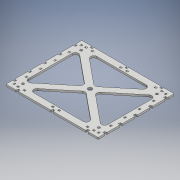
# Autodesk Inventor part: turtlebot_installation_top
Saved by Autodesk Inventor 2018 (Build 220112000, 112)
## iProperties
Created: 2018-07-16
Part Number: turtlebot_installation_top
Material: Generic
Document SubType Name: Modeling
Designer: Tsche
Density: 1 g/cm^3
Appearance: Default
Author: Tsche
Autodesk Inventor part; units mm, degrees
ref_plane "YZ Plane" through (0, 0, 0) normal (1, 0, 0) x (0, 1, 0)
ref_plane "XZ Plane" through (0, 0, 0) normal (0, 1, 0) x (-1, 0, 0)
ref_plane "XY Plane" through (0, 0, 0) normal (0, 0, 1) x (1, 0, 0)
sketch "Sketch1" plane through (0, 0, 0) normal (0, 0, 1) x (1, 0, 0)
  line L0 (-73, 60) -> (-73, 49.6)
  line L1 (-73, -60) -> (0, 0) construction
  line L2 (-73, -1.6) -> (-69.9, -1.6)
  line L3 (-69.9, -1.6) -> (-69.9, 1.6)
  line L4 (-69.9, 1.6) -> (-73, 1.6)
  line L5 (-73, 1.6) -> (-73, -1.6) construction
  line L6 (-73, -1.6) -> (-73, -22.4)
  line L7 (-73, 0) -> (-69.9, 0) construction
  line L8 (-102.2, 0) -> (102.2, 0) construction
  line L9 (0, 84) -> (0, -84) construction
  line L10 (-73, -25.6) -> (-69.9, -25.6)
  line L11 (-69.9, -25.6) -> (-69.9, -22.4)
  line L12 (-69.9, -22.4) -> (-73, -22.4)
  line L13 (-73, 49.6) -> (-69.9, 49.6)
  line L14 (-69.9, 49.6) -> (-69.9, 46.4)
  line L15 (-69.9, 46.4) -> (-73, 46.4)
  line L16 (-73, 49.6) -> (-73, 46.4) construction
  line L17 (-73, 46.4) -> (-73, 25.6)
  line L18 (-73, -22.4) -> (-73, -25.6) construction
  line L19 (-73, -25.6) -> (-73, -46.4)
  line L20 (-73, -24) -> (-69.9, -24) construction
  line L21 (-73, 48) -> (-69.9, 48) construction
  line L22 (-73, -49.6) -> (-69.9, -49.6)
  line L23 (-69.9, -49.6) -> (-69.9, -46.4)
  line L24 (-69.9, -46.4) -> (-73, -46.4)
  line L25 (-73, -46.4) -> (-73, -49.6) construction
  line L26 (-73, -49.6) -> (-73, -60)
  line L27 (-73, -48) -> (-69.9, -48) construction
  line L28 (-73, 22.4) -> (-69.9, 22.4)
  line L29 (-69.9, 22.4) -> (-69.9, 25.6)
  line L30 (-69.9, 25.6) -> (-73, 25.6)
  line L31 (-73, 25.6) -> (-73, 22.4) construction
  line L32 (-73, 22.4) -> (-73, 1.6)
  line L33 (-73, 24) -> (-69.9, 24) construction
  line L34 (0, 60) -> (-1.5, 60) construction
  line L35 (0, 0) -> (-73, 60) construction
  line L36 (-67, -10) -> (-65.7, -10)
  line L37 (-65.7, -10) -> (-65.7, -13)
  line L38 (-65.7, -13) -> (-67, -13)
  line L39 (-67, -13) -> (-67, -10)
  line L40 (-67, -11.5) -> (-65.7, -11.5) construction
  line L41 (-65.7, -35.5) -> (-67, -35.5)
  line L42 (-67, -34) -> (-65.7, -34) construction
  line L43 (-67, -35.5) -> (-67, -32.5)
  line L44 (-67, -32.5) -> (-65.7, -32.5)
  line L45 (-65.7, -32.5) -> (-65.7, -35.5)
  line L46 (-67, -51.5) -> (-65.7, -51.5)
  line L47 (-67, -53) -> (-65.7, -53) construction
  line L48 (-65.7, -51.5) -> (-65.7, -54.5)
  line L49 (-67, -54.5) -> (-67, -51.5)
  line L50 (-65.7, -54.5) -> (-67, -54.5)
  line L51 (-67, 10) -> (-65.7, 10)
  line L52 (-65.7, 10) -> (-65.7, 13)
  line L53 (-65.7, 13) -> (-67, 13)
  line L54 (-67, 13) -> (-67, 10)
  line L55 (-67, 11.5) -> (-65.7, 11.5) construction
  line L56 (-65.7, 35.5) -> (-67, 35.5)
  line L57 (-67, 34) -> (-65.7, 34) construction
  line L58 (-67, 35.5) -> (-67, 32.5)
  line L59 (-67, 32.5) -> (-65.7, 32.5)
  line L60 (-65.7, 32.5) -> (-65.7, 35.5)
  line L61 (-67, 51.5) -> (-65.7, 51.5)
  line L62 (-67, 53) -> (-65.7, 53) construction
  line L63 (-65.7, 51.5) -> (-65.7, 54.5)
  line L64 (-67, 54.5) -> (-67, 51.5)
  line L65 (-65.7, 54.5) -> (-67, 54.5)
  line L66 (73, 60) -> (73, 49.6)
  line L67 (73, -60) -> (0, 0) construction
  line L68 (73, -1.6) -> (69.9, -1.6)
  line L69 (69.9, -1.6) -> (69.9, 1.6)
  line L70 (69.9, 1.6) -> (73, 1.6)
  line L71 (73, 1.6) -> (73, -1.6) construction
  line L72 (73, -1.6) -> (73, -22.4)
  line L73 (73, 0) -> (69.9, 0) construction
  line L74 (73, -25.6) -> (69.9, -25.6)
  line L75 (69.9, -25.6) -> (69.9, -22.4)
  line L76 (69.9, -22.4) -> (73, -22.4)
  line L77 (73, 49.6) -> (69.9, 49.6)
  line L78 (69.9, 49.6) -> (69.9, 46.4)
  line L79 (69.9, 46.4) -> (73, 46.4)
  line L80 (73, 49.6) -> (73, 46.4) construction
  line L81 (73, 46.4) -> (73, 25.6)
  line L82 (73, -22.4) -> (73, -25.6) construction
  line L83 (73, -25.6) -> (73, -46.4)
  line L84 (73, -24) -> (69.9, -24) construction
  line L85 (73, 48) -> (69.9, 48) construction
  line L86 (73, -49.6) -> (69.9, -49.6)
  line L87 (69.9, -49.6) -> (69.9, -46.4)
  line L88 (69.9, -46.4) -> (73, -46.4)
  line L89 (73, -46.4) -> (73, -49.6) construction
  line L90 (73, -49.6) -> (73, -60)
  line L91 (73, -48) -> (69.9, -48) construction
  line L92 (73, 22.4) -> (69.9, 22.4)
  line L93 (69.9, 22.4) -> (69.9, 25.6)
  line L94 (69.9, 25.6) -> (73, 25.6)
  line L95 (73, 25.6) -> (73, 22.4) construction
  line L96 (73, 22.4) -> (73, 1.6)
  line L97 (73, 24) -> (69.9, 24) construction
  line L98 (0, 0) -> (73, 60) construction
  line L99 (67, -10) -> (65.7, -10)
  line L100 (65.7, -10) -> (65.7, -13)
  line L101 (65.7, -13) -> (67, -13)
  line L102 (67, -13) -> (67, -10)
  line L103 (67, -11.5) -> (65.7, -11.5) construction
  line L104 (65.7, -35.5) -> (67, -35.5)
  line L105 (67, -34) -> (65.7, -34) construction
  line L106 (67, -35.5) -> (67, -32.5)
  line L107 (67, -32.5) -> (65.7, -32.5)
  line L108 (65.7, -32.5) -> (65.7, -35.5)
  line L109 (67, -51.5) -> (65.7, -51.5)
  line L110 (67, -53) -> (65.7, -53) construction
  line L111 (65.7, -51.5) -> (65.7, -54.5)
  line L112 (67, -54.5) -> (67, -51.5)
  line L113 (65.7, -54.5) -> (67, -54.5)
  line L114 (67, 10) -> (65.7, 10)
  line L115 (67, 11.5) -> (65.7, 11.5) construction
  line L116 (67, 13) -> (67, 10)
  line L117 (65.7, 10) -> (65.7, 13)
  line L118 (65.7, 13) -> (67, 13)
  line L119 (67, 51.5) -> (65.7, 51.5)
  line L120 (67, 53) -> (65.7, 53) construction
  line L121 (67, 54.5) -> (67, 51.5)
  line L122 (65.7, 51.5) -> (65.7, 54.5)
  line L123 (65.7, 54.5) -> (67, 54.5)
  line L124 (67, 32.5) -> (65.7, 32.5)
  line L125 (67, 34) -> (65.7, 34) construction
  line L126 (67, 35.5) -> (67, 32.5)
  line L127 (65.7, 32.5) -> (65.7, 35.5)
  line L128 (65.7, 35.5) -> (67, 35.5)
  line L129 (-63, 45.3087) -> (-63, -45.3087)
  line L130 (-63, -45.3087) -> (-7.8744, 0)
  line L131 (-63, 45.3087) -> (-7.8744, 0)
  line L132 (-52.9589, 50) -> (0, 6.4721)
  line L133 (52.9589, 50) -> (0, 6.4721)
  line L134 (-52.9589, 50) -> (52.9589, 50)
  line L135 (63, 45.3087) -> (63, -45.3087)
  line L136 (63, -45.3087) -> (7.8744, 0)
  line L137 (63, 45.3087) -> (7.8744, 0)
  line L138 (-52.9589, -50) -> (0, -6.4721)
  line L139 (52.9589, -50) -> (0, -6.4721)
  line L140 (-52.9589, -50) -> (52.9589, -50)
  line L141 (-1.5, 60) -> (-1.5, 56.9)
  line L142 (-1.5, 56.9) -> (0, 56.9)
  line L143 (-1.5, 60) -> (-53.4, 60)
  line L144 (-56.6, 60) -> (-56.6, 56.9)
  line L145 (-56.6, 56.9) -> (-53.4, 56.9)
  line L146 (-53.4, 56.9) -> (-53.4, 60)
  line L147 (-56.6, 60) -> (-73, 60)
  line L148 (-53.4, 60) -> (-56.6, 60) construction
  line L149 (-55, 56.9) -> (-55, 60) construction
  line L150 (-3.5, 54) -> (-6.5, 54)
  line L151 (-6.5, 54) -> (-6.5, 52.7)
  line L152 (-6.5, 52.7) -> (-3.5, 52.7)
  line L153 (-3.5, 52.7) -> (-3.5, 54)
  line L154 (-5, 54) -> (-5, 52.7) construction
  line L155 (-48.5, 52.7) -> (-48.5, 54)
  line L156 (-50, 54) -> (-50, 52.7) construction
  line L157 (-51.5, 54) -> (-51.5, 52.7)
  line L158 (-48.5, 54) -> (-51.5, 54)
  line L159 (-51.5, 52.7) -> (-48.5, 52.7)
  line L160 (-61.5, 52.7) -> (-61.5, 54)
  line L161 (-60, 54) -> (-60, 52.7) construction
  line L162 (-58.5, 54) -> (-58.5, 52.7)
  line L163 (-61.5, 54) -> (-58.5, 54)
  line L164 (-58.5, 52.7) -> (-61.5, 52.7)
  line L165 (0, -60) -> (-1.5, -60) construction
  line L166 (-1.5, -60) -> (-1.5, -56.9)
  line L167 (-1.5, -56.9) -> (0, -56.9)
  line L168 (-1.5, -60) -> (-53.4, -60)
  line L169 (-56.6, -60) -> (-56.6, -56.9)
  line L170 (-56.6, -56.9) -> (-53.4, -56.9)
  line L171 (-53.4, -56.9) -> (-53.4, -60)
  line L172 (-56.6, -60) -> (-73, -60)
  line L173 (-53.4, -60) -> (-56.6, -60) construction
  line L174 (-55, -56.9) -> (-55, -60) construction
  line L175 (-3.5, -54) -> (-6.5, -54)
  line L176 (-6.5, -54) -> (-6.5, -52.7)
  line L177 (-6.5, -52.7) -> (-3.5, -52.7)
  line L178 (-3.5, -52.7) -> (-3.5, -54)
  line L179 (-5, -54) -> (-5, -52.7) construction
  line L180 (-48.5, -52.7) -> (-48.5, -54)
  line L181 (-50, -54) -> (-50, -52.7) construction
  line L182 (-51.5, -54) -> (-51.5, -52.7)
  line L183 (-48.5, -54) -> (-51.5, -54)
  line L184 (-51.5, -52.7) -> (-48.5, -52.7)
  line L185 (-58.5, -54) -> (-58.5, -52.7)
  line L186 (-60, -54) -> (-60, -52.7) construction
  line L187 (-58.5, -52.7) -> (-61.5, -52.7)
  line L188 (-61.5, -52.7) -> (-61.5, -54)
  line L189 (-61.5, -54) -> (-58.5, -54)
  line L190 (0, -60) -> (1.5, -60) construction
  line L191 (61.5, -52.7) -> (61.5, -54)
  line L192 (58.5, -52.7) -> (61.5, -52.7)
  line L193 (60, -54) -> (60, -52.7) construction
  line L194 (58.5, -54) -> (58.5, -52.7)
  line L195 (56.6, -60) -> (73, -60)
  line L196 (61.5, -54) -> (58.5, -54)
  line L197 (6.5, -52.7) -> (3.5, -52.7)
  line L198 (3.5, -52.7) -> (3.5, -54)
  line L199 (5, -54) -> (5, -52.7) construction
  line L200 (6.5, -54) -> (6.5, -52.7)
  line L201 (3.5, -54) -> (6.5, -54)
  line L202 (1.5, -56.9) -> (0, -56.9)
  line L203 (1.5, -60) -> (1.5, -56.9)
  line L204 (1.5, -60) -> (53.4, -60)
  line L205 (56.6, -60) -> (56.6, -56.9)
  line L206 (55, -56.9) -> (55, -60) construction
  line L207 (56.6, -56.9) -> (53.4, -56.9)
  line L208 (53.4, -60) -> (56.6, -60) construction
  line L209 (51.5, -54) -> (51.5, -52.7)
  line L210 (50, -54) -> (50, -52.7) construction
  line L211 (48.5, -52.7) -> (48.5, -54)
  line L212 (51.5, -52.7) -> (48.5, -52.7)
  line L213 (48.5, -54) -> (51.5, -54)
  line L214 (53.4, -56.9) -> (53.4, -60)
  line L215 (0, 60) -> (1.5, 60) construction
  line L216 (1.5, 60) -> (1.5, 56.9)
  line L217 (1.5, 56.9) -> (0, 56.9)
  line L218 (1.5, 60) -> (53.4, 60)
  line L219 (56.6, 60) -> (56.6, 56.9)
  line L220 (56.6, 56.9) -> (53.4, 56.9)
  line L221 (53.4, 56.9) -> (53.4, 60)
  line L222 (56.6, 60) -> (73, 60)
  line L223 (53.4, 60) -> (56.6, 60) construction
  line L224 (55, 56.9) -> (55, 60) construction
  line L225 (3.5, 54) -> (6.5, 54)
  line L226 (6.5, 54) -> (6.5, 52.7)
  line L227 (6.5, 52.7) -> (3.5, 52.7)
  line L228 (3.5, 52.7) -> (3.5, 54)
  line L229 (5, 54) -> (5, 52.7) construction
  line L230 (48.5, 52.7) -> (48.5, 54)
  line L231 (50, 54) -> (50, 52.7) construction
  line L232 (51.5, 54) -> (51.5, 52.7)
  line L233 (48.5, 54) -> (51.5, 54)
  line L234 (51.5, 52.7) -> (48.5, 52.7)
  line L235 (58.5, 54) -> (58.5, 52.7)
  line L236 (60, 54) -> (60, 52.7) construction
  line L237 (58.5, 52.7) -> (61.5, 52.7)
  line L238 (61.5, 52.7) -> (61.5, 54)
  line L239 (61.5, 54) -> (58.5, 54)
  circle A0 centre (0, 0) radius 3.15
  circle A1 centre (-60, -46) radius 1.85
  circle A2 centre (60, -46) radius 1.85
  circle A3 centre (-60, 46) radius 1.85
  circle A4 centre (60, 46) radius 1.85
  dimension "d0" = 120
  dimension "d2" = 3.1
  dimension "d3" = 3.2
  dimension "d4" = 24
  dimension "d5" = 24
  dimension "d6" = 24
  dimension "d7" = 24
  dimension "d8" = 73
  dimension "d9" = 3
  dimension "d10" = 1.3
  dimension "d11" = 11.5
  dimension "d12" = 6
  dimension "d15" = 22.5
  dimension "d22" = 41.5
  dimension "d33" = 10
  dimension "d34" = 5
  dimension "d35" = 5
  dimension "d36" = 5
  dimension "d37" = 10
  dimension "d38" = 10
  dimension "d39" = 1.5
  dimension "d40" = 18
  dimension "d41" = 6
  dimension "d42" = 5
  dimension "d45" = 45
  dimension "d50" = 5
  dimension "d52" = 6.3
  dimension "d53" = 3.7
  dimension "d54" = 60
  dimension "d55" = 46
  constraints: 476 end point, 182 symmetric about line, 40 perpendicular, 17 midpoint, 15 point on line, 8 equal length, 8 horizontal, 6 collinear, 6 parallel, 5 centre point, 5 vertical, 1 coincident, 36 other
  measures "d0" distance of L0.start L1.start
  measures "d2" distance of L3.end L4.end
  measures "d3" distance of L2.end L3.end
  measures "d4" distance between parallel lines of L8 L20
  measures "d5" distance between parallel lines of L20 L27
  measures "d6" distance between parallel lines of L8 L33
  measures "d7" distance from line of L21.start L33
  measures "d8" distance between parallel lines of L9 L26
  measures "d9" distance of L36.end L37.end
  measures "d10" distance of L37.end L38.end
  measures "d11" distance between parallel lines of L7 L40
  measures "d12" distance between parallel lines of L6 L39
  measures "d15" distance of L38.end L41.end
  measures "d22" distance of L36.end L46.end
  measures "d33" distance between parallel lines of L20 L42
  measures "d34" distance between parallel lines of L27 L47
  measures "d35" distance between parallel lines of L132 L35
  measures "d36" distance between parallel lines of L35 L131
  measures "d37" distance between parallel lines of L32 L129
  measures "d38" distance between parallel lines of L34 L134
  measures "d39" distance of L141.end L142.end
  measures "d40" distance between parallel lines of L0 L149
  measures "d41" distance between parallel lines of L143 L150
  measures "d42" distance between parallel lines of L9 L154
  measures "d45" distance of L152.end L155.start
  measures "d50" distance between parallel lines of L149 L156
  measures "d52" diameter of A0
  measures "d53" diameter of A1
  measures "d54" distance from line of L9 A1.centre
  measures "d55" distance from line of L8 A1.centre
extrude "Extrusion1" add sketch "Sketch1" along normal blind 3
fillet "Fillet1" radius 1 36 edges at (-73, -60, 1.5) (-73, -49.6, 1.5) (-73, -46.4, 1.5) (-73, -22.4, 1.5) (-73, -25.6, 1.5) (-73, 1.6, 1.5) (-73, -1.6, 1.5) (-73, 25.6, 1.5) (-73, 22.4, 1.5) (-73, 49.6, 1.5) (-73, 46.4, 1.5) (-73, 60, 1.5) (73, -60, 1.5) (73, -49.6, 1.5) (73, -46.4, 1.5) (73, -25.6, 1.5) (73, -22.4, 1.5) (73, -1.6, 1.5) (73, 1.6, 1.5) (73, 22.4, 1.5) (73, 25.6, 1.5) (73, 46.4, 1.5) (73, 49.6, 1.5) (73, 60, 1.5) (-56.6, -60, 1.5) (-53.4, -60, 1.5) (-1.5, -60, 1.5) (1.5, -60, 1.5) (53.4, -60, 1.5) (56.6, -60, 1.5) (-1.5, 60, 1.5) (1.5, 60, 1.5) (53.4, 60, 1.5) (56.6, 60, 1.5) (-53.4, 60, 1.5) (-56.6, 60, 1.5)
chamfer "Chamfer1" distance 1 angle 45 48 edges at (-67, -34, 3) (-67, -53, 3) (-67, -53, 0) (-67, -34, 0) (-67, -11.5, 3) (-67, -11.5, 0) (-67, 11.5, 3) (-67, 11.5, 0) (-67, 34, 3) (-67, 34, 0) (-67, 53, 3) (-67, 53, 0) (67, -53, 3) (67, -53, 0) (67, -34, 3) (67, -34, 0) (67, -11.5, 3) (67, -11.5, 0) (67, 11.5, 3) (67, 11.5, 0) (67, 34, 3) (67, 34, 0) (67, 53, 3) (67, 53, 0) (-60, -54, 3) (-60, -54, 0) (-50, -54, 3) (-50, -54, 0) (-5, -54, 3) (-5, -54, 0) (5, -54, 3) (50, -54, 3) (50, -54, 0) (5, -54, 0) (60, -54, 3) (60, -54, 0) (50, 54, 0) (50, 54, 3) (60, 54, 0) (60, 54, 3) (5, 54, 0) (5, 54, 3) (-5, 54, 0) (-5, 54, 3) (-50, 54, 0) (-50, 54, 3) (-60, 54, 0) (-60, 54, 3)
fillet "Fillet2" radius 5 12 edges at (63, 45.3087, 1.5) (52.9589, 50, 1.5) (-52.9589, 50, 1.5) (-63, 45.3087, 1.5) (0, 6.4721, 1.5) (-7.8744, 0, 1.5) (0, -6.4721, 1.5) (7.8744, 0, 1.5) (-63, -45.3087, 1.5) (-52.9589, -50, 1.5) (52.9589, -50, 1.5) (63, -45.3087, 1.5)
body "Solid1"
